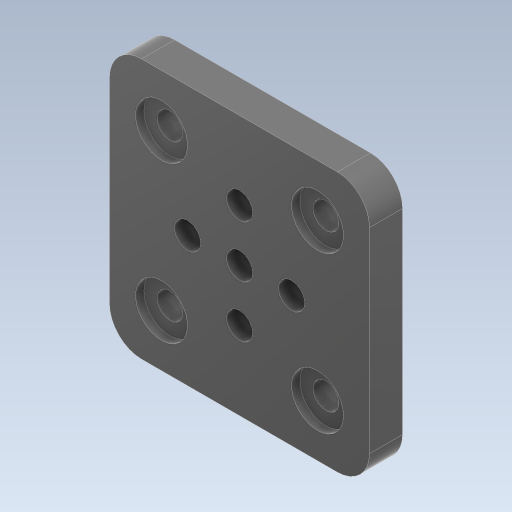
# Autodesk Inventor part: vwheel_plate
Saved by Autodesk Inventor 2023 (Build 270158000, 158)
## iProperties
Created: 2023-01-20
Part Number: vwheel_plate
Material: Aluminum 6061
Document SubType Name: Modeling
Designer: adars
Density: 2.7 g/cm^3
Appearance: Anodized - Black
Author: adars
Autodesk Inventor part; units mm, degrees
ref_plane "YZ Plane" through (0, 0, 0) normal (1, 0, 0) x (0, 1, 0)
ref_plane "XZ Plane" through (0, 0, 0) normal (0, 1, 0) x (-1, 0, 0)
ref_plane "XY Plane" through (0, 0, 0) normal (0, 0, 1) x (1, 0, 0)
sketch "Sketch1" plane through (0, 0, 0) normal (0, 0, 1) x (1, 0, 0)
  line L0 (-18.83, -25) -> (18.83, -25)
  line L1 (25, -18.83) -> (25, 18.83)
  line L2 (18.83, 25) -> (-18.83, 25)
  line L3 (-25, 18.83) -> (-25, -18.83)
  line L4 (-25, -25) -> (25, 25) construction
  line L5 (25, -25) -> (-25, 25) construction
  circle A0 centre (0, 0) radius 2.51
  circle A1 centre (0, 10) radius 2.51
  circle A2 centre (-10, 0) radius 2.51
  circle A3 centre (0, -10) radius 2.51
  circle A4 centre (10, 0) radius 2.51
  arc A5 (-18.83, 25) -> (-25, 18.83) centre (-18.83, 18.83) ccw
  arc A6 (25, 18.83) -> (18.83, 25) centre (18.83, 18.83) ccw
  arc A7 (18.83, -25) -> (25, -18.83) centre (18.83, -18.83) ccw
  arc A8 (-25, -18.83) -> (-18.83, -25) centre (-18.83, -18.83) ccw
  dimension "d0" = 50
  dimension "d1" = 50
  dimension "d2" = 5.02
  dimension "d3" = 5.02
  dimension "d6" = 360
  dimension "d8" = 10
  dimension "d9" = 6.17
  constraints: 12 end point, 9 centre point, 8 point on circle, 8 point on line, 8 tangent, 3 equal radius, 2 midpoint, 2 parallel, 1 coincident, 1 horizontal, 1 perpendicular, 9 other
  measures "d0" distance of L5.end L4.end
  measures "d1" distance of L4.end L5.start
  measures "d2" diameter of A0
  measures "d3" diameter of A1
  measures "d8" distance of A1.centre point (0, 0)
  measures "d9" radius of A5
extrude "Extrusion1" add sketch "Sketch1" along normal mid plane 6.35
sketch "Sketch2" plane through (0, 0, 3.175) normal (0, 0, 1) x (1, 0, 0)
  circle A0 centre (15, 15) radius 5
  circle A1 centre (15, 15) radius 2.5
  point P0 (0, 0)
  dimension "d18" = 10
  dimension "d19" = 5
  dimension "d20" = 15
  dimension "d21" = 15
  constraints: 2 centre point, 1 coincident
  measures "d18" diameter of A0
  measures "d19" diameter of A1
  measures "d20" horizontal distance of point (0, 0) A0.centre
  measures "d21" horizontal distance of point (0, 0) A0.centre
extrude "Extrusion3" cut sketch "Sketch2" against normal blind 1.625 contours A0 | A1
extrude "Extrusion4" cut sketch "Sketch2" against normal through all contours A1
mirror "Mirror1" about plane through (0, 0, 0) normal (1, 0, 0) of "Extrusion3", "Extrusion4"
mirror "Mirror2" about plane through (0, 0, 0) normal (0, 1, 0) of "Extrusion3", "Extrusion4", "Mirror1"
body "Solid1"
